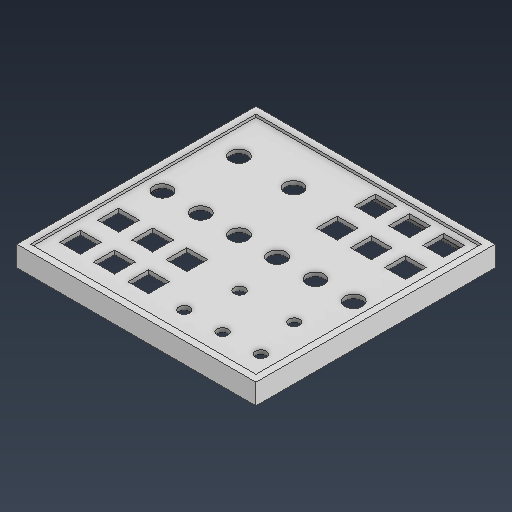
# Autodesk Inventor part: Faceplate
Saved by Autodesk Inventor 2025.3 (Build 293356000, 356)
## iProperties
Created: 2025-09-08
Part Number: Faceplate
Material: Generic
Document SubType Name: Modeling
Designer: tolga
Density: 1 g/cm^3
Appearance: Default
Author: tolga
Autodesk Inventor part; units mm, degrees
ref_plane "YZ Plane" through (0, 0, 0) normal (1, 0, 0) x (0, 1, 0)
ref_plane "XZ Plane" through (0, 0, 0) normal (0, 1, 0) x (-1, 0, 0)
ref_plane "XY Plane" through (0, 0, 0) normal (0, 0, 1) x (1, 0, 0)
sketch "Sketch1" plane through (0, 0, 0) normal (0, 1, 0) x (-1, 0, 0)
  line L0 (0, 0) -> (-175, 0)
  line L1 (-175, 0) -> (-175, -175)
  line L2 (-175, -175) -> (0, -175)
  line L3 (0, -175) -> (0, 0)
  dimension "d0" = 175
  dimension "d1" = 175
  constraints: 8 end point, 2 parallel, 1 horizontal, 1 perpendicular
  measures "d0" distance of L2.end L1.end
  measures "d1" distance of L1.end L0.end
extrude "Extrusion1" add sketch "Sketch1" along normal blind 3
sketch "Sketch2" plane through (0, 3, 0) normal (0, 1, 0) x (1, 0, 0)
  line L0 (175, 0) -> (175, 175) projected
  line L1 (175, 175) -> (0, 175) projected
  line L2 (0, 175) -> (0, 0) projected
  line L3 (0, 0) -> (175, 0) projected
  line L4 (5, 5) -> (5, 170)
  line L5 (5, 170) -> (170, 170)
  line L6 (170, 170) -> (170, 5)
  line L7 (170, 5) -> (5, 5)
  dimension "d4" = 5
  constraints: 8 end point, 3 other
  measures "d4" distance between parallel lines of L2 L4
extrude "Extrusion2" add sketch "Sketch2" along normal blind 2
sketch "Sketch3" plane through (0, 3, 0) normal (0, 1, 0) x (1, 0, 0)
  line L0 (5, 5) -> (170, 5) construction
  line L1 (170, 5) -> (170, 170) construction
  line L2 (170, 170) -> (5, 170) construction
  line L3 (5, 170) -> (5, 5) construction
  line L4 (6, 66) -> (84, 66) construction
  line L5 (84, 66) -> (84, 6) construction
  line L6 (84, 6) -> (6, 6) construction
  line L7 (6, 6) -> (6, 66) construction
  line L8 (91, 109) -> (169, 109) construction
  line L9 (169, 109) -> (169, 169) construction
  line L10 (169, 169) -> (91, 169) construction
  line L11 (91, 169) -> (91, 109) construction
  line L12 (6, 169) -> (81, 169) construction
  line L13 (81, 169) -> (81, 104) construction
  line L14 (6, 74) -> (6, 169) construction
  line L15 (6, 74) -> (169, 74) construction
  line L16 (169, 74) -> (169, 104) construction
  line L17 (169, 104) -> (81, 104) construction
  line L18 (89, 69) -> (169, 69) construction
  line L19 (169, 69) -> (169, 39) construction
  line L20 (169, 39) -> (89, 39) construction
  line L21 (89, 39) -> (89, 69) construction
  line L22 (89, 34) -> (169, 34) construction
  line L23 (169, 34) -> (169, 9) construction
  line L24 (169, 9) -> (89, 9) construction
  line L25 (89, 9) -> (89, 34) construction
  line L26 (12.4, 34) -> (27.6, 34)
  line L27 (27.6, 34) -> (27.6, 18.8)
  line L28 (27.6, 18.8) -> (12.4, 18.8)
  line L29 (12.4, 18.8) -> (12.4, 34)
  line L30 (12.4, 62) -> (27.6, 62)
  line L31 (12.4, 46.8) -> (12.4, 62)
  line L32 (27.6, 46.8) -> (12.4, 46.8)
  line L33 (27.6, 62) -> (27.6, 46.8)
  line L34 (37.4, 34) -> (52.6, 34)
  line L35 (37.4, 18.8) -> (37.4, 34)
  line L36 (52.6, 18.8) -> (37.4, 18.8)
  line L37 (52.6, 34) -> (52.6, 18.8)
  line L38 (37.4, 62) -> (52.6, 62)
  line L39 (37.4, 46.8) -> (37.4, 62)
  line L40 (52.6, 46.8) -> (37.4, 46.8)
  line L41 (52.6, 62) -> (52.6, 46.8)
  line L42 (62.4, 34) -> (77.6, 34)
  line L43 (62.4, 18.8) -> (62.4, 34)
  line L44 (77.6, 18.8) -> (62.4, 18.8)
  line L45 (77.6, 34) -> (77.6, 18.8)
  line L46 (62.4, 62) -> (77.6, 62)
  line L47 (62.4, 46.8) -> (62.4, 62)
  line L48 (77.6, 46.8) -> (62.4, 46.8)
  line L49 (77.6, 62) -> (77.6, 46.8)
  line L50 (12.4, 62) -> (12.4, 18.8) construction
  line L51 (12.4, 62) -> (77.6, 62) construction
  line L52 (97.4, 137) -> (112.6, 137)
  line L53 (112.6, 137) -> (112.6, 121.8)
  line L54 (112.6, 121.8) -> (97.4, 121.8)
  line L55 (97.4, 121.8) -> (97.4, 137)
  line L56 (97.4, 165) -> (112.6, 165)
  line L57 (97.4, 149.8) -> (97.4, 165)
  line L58 (112.6, 149.8) -> (97.4, 149.8)
  line L59 (112.6, 165) -> (112.6, 149.8)
  line L60 (122.4, 137) -> (137.6, 137)
  line L61 (122.4, 121.8) -> (122.4, 137)
  line L62 (137.6, 121.8) -> (122.4, 121.8)
  line L63 (137.6, 137) -> (137.6, 121.8)
  line L64 (122.4, 165) -> (137.6, 165)
  line L65 (122.4, 149.8) -> (122.4, 165)
  line L66 (137.6, 149.8) -> (122.4, 149.8)
  line L67 (137.6, 165) -> (137.6, 149.8)
  line L68 (147.4, 137) -> (162.6, 137)
  line L69 (147.4, 121.8) -> (147.4, 137)
  line L70 (162.6, 121.8) -> (147.4, 121.8)
  line L71 (162.6, 137) -> (162.6, 121.8)
  line L72 (147.4, 165) -> (162.6, 165)
  line L73 (147.4, 149.8) -> (147.4, 165)
  line L74 (162.6, 149.8) -> (147.4, 149.8)
  line L75 (162.6, 165) -> (162.6, 149.8)
  line L76 (97.4, 165) -> (97.4, 121.8) construction
  line L77 (97.4, 165) -> (162.6, 165) construction
  circle A0 centre (109, 54) radius 12.5 construction
  circle A1 centre (149, 54) radius 12.5 construction
  circle A2 centre (109, 54) radius 4
  circle A3 centre (149, 54) radius 4
  circle A4 centre (101, 21.5) radius 8.1 construction
  circle A5 centre (129, 21.5) radius 8.1 construction
  circle A6 centre (157, 21.5) radius 8.1 construction
  circle A7 centre (101, 21.5) radius 4
  circle A8 centre (129, 21.5) radius 4
  circle A9 centre (157, 21.5) radius 4
  circle A10 centre (157.5, 89) radius 6.5
  circle A11 centre (129.5, 89) radius 6.5
  circle A12 centre (101.5, 89) radius 6.5
  circle A13 centre (73.5, 89) radius 6.5
  circle A14 centre (45.5, 89) radius 6.5
  circle A15 centre (17.5, 89) radius 6.5
  circle A16 centre (63.5, 139) radius 6.5
  circle A17 centre (23.5, 139) radius 6.5
  point P0 (0, 0)
  point P1 (6, 36)
  point P2 (45, 62)
  point P3 (45, 66)
  point P4 (20, 46.8)
  point P5 (27.6, 54.4)
  point P6 (130, 165)
  point P7 (105, 149.8)
  point P8 (112.6, 157.4)
  point P9 (130, 165)
  point P10 (130, 109)
  point P11 (89, 54)
  point P12 (169, 21.5)
  point P13 (169, 89)
  point P14 (81, 136.5)
  dimension "d7" = 1
  dimension "d8" = 1
  dimension "d9" = 60
  dimension "d10" = 78
  dimension "d11" = 78
  dimension "d12" = 60
  dimension "d13" = 1
  dimension "d14" = 1
  dimension "d15" = 1
  dimension "d16" = 1
  dimension "d17" = 75
  dimension "d19" = 1
  dimension "d20" = 5
  dimension "d21" = 30
  dimension "d22" = 5
  dimension "d23" = 5
  dimension "d24" = 1
  dimension "d27" = 5
  dimension "d28" = 5
  dimension "d29" = 1
  dimension "d30" = 4
  dimension "d31" = 25
  dimension "d32" = 15.2
  dimension "d33" = 15.2
  dimension "d37" = 28
  dimension "d40" = 25
  dimension "d43" = 12.8
  dimension "d44" = 6.4
  dimension "d45" = 4
  dimension "d46" = 14
  dimension "d47" = 11.6
  dimension "d52" = 15.2
  dimension "d53" = 15.2
  dimension "d54" = 28
  dimension "d55" = 25
  dimension "d56" = 12.8
  dimension "d57" = 30
  dimension "d58" = 80
  dimension "d59" = 25
  dimension "d60" = 25
  dimension "d61" = 20
  dimension "d62" = 40
  dimension "d63" = 8
  dimension "d64" = 8
  dimension "d67" = 80
  dimension "d68" = 16.2
  dimension "d69" = 16.2
  dimension "d70" = 16.2
  dimension "d71" = 28
  dimension "d72" = 28
  dimension "d73" = 12
  dimension "d74" = 8
  dimension "d75" = 8
  dimension "d76" = 8
  dimension "d77" = 13
  dimension "d80" = 28
  dimension "d85" = 11.5
  dimension "d86" = 163
  dimension "d87" = 65
  dimension "d88" = 95
  dimension "d89" = 88
  dimension "d90" = 13
  dimension "d91" = 13
  dimension "d92" = 30
  constraints: 148 end point, 18 centre point, 14 midpoint, 13 parallel, 11 horizontal, 11 perpendicular, 7 horizontal alignment, 6 collinear, 5 coincident, 2 vertical, 2 vertical alignment, 86 other
  measures "d7" distance between parallel lines of L7 L3
  measures "d8" distance between parallel lines of L0 L6
  measures "d9" distance between parallel lines of L6 L4
  measures "d10" distance between parallel lines of L7 L5
  measures "d11" distance of L10.end L9.end
  measures "d12" distance of L9.end L8.end
  measures "d13" distance between parallel lines of L2 L10
  measures "d14" distance between parallel lines of L1 L9
  measures "d15" distance between parallel lines of L2 L12
  measures "d16" distance between parallel lines of L3 L14
  measures "d17" distance between parallel lines of L14 L13
  measures "d19" distance between parallel lines of L1 L16
  measures "d20" distance between parallel lines of L8 L17
  measures "d21" distance between parallel lines of L17 L15
  measures "d22" distance between parallel lines of L15 L18
  measures "d23" distance between parallel lines of L5 L21
  measures "d24" distance between parallel lines of L1 L19
  measures "d27" distance between parallel lines of L5 L25
  measures "d28" distance between parallel lines of L20 L22
  measures "d29" distance between parallel lines of L1 L23
  measures "d30" distance between parallel lines of L0 L24
  measures "d31" distance between parallel lines of L24 L22
  measures "d32" distance of L27.end L28.end
  measures "d33" distance of L26.end L27.end
  measures "d37" distance of L27.end L32.start
  measures "d40" distance of L27.end L36.start
  measures "d43" distance between parallel lines of L6 L28
  measures "d44" distance between parallel lines of L7 L31
  measures "d45" distance between parallel lines of L4 L51
  measures "d46" distance from line of L7 point (20, 46.8)
  measures "d47" distance from line of L4 point (27.6, 54.4)
  measures "d52" distance of L53.end L76.end
  measures "d53" distance of L53.start L53.end
  measures "d54" distance of L53.end L58.start
  measures "d55" distance of L53.end L62.start
  measures "d56" distance between parallel lines of L8 L54
  measures "d57" distance between parallel lines of L18 L20
  measures "d58" distance between parallel lines of L19 L21
  measures "d59" diameter of A0
  measures "d60" diameter of A1
  measures "d61" distance from line of L21 A0.centre
  measures "d62" distance of A0.centre A1.centre
  measures "d63" diameter of A2
  measures "d64" diameter of A3
  measures "d67" distance between parallel lines of L23 L25
  measures "d68" diameter of A4
  measures "d69" diameter of A5
  measures "d70" diameter of A6
  measures "d71" distance of A5.centre A4.centre
  measures "d72" distance of A6.centre A5.centre
  measures "d73" distance from line of L25 A4.centre
  measures "d74" diameter of A7
  measures "d75" diameter of A8
  measures "d76" diameter of A9
  measures "d77" diameter of A10
  measures "d80" distance of A10.centre A11.centre
  measures "d85" distance from line of L16 A10.centre
  measures "d86" distance of L14.start L15.end
  measures "d87" distance of L12.end L13.end
  measures "d88" distance of L14.start L12.start
  measures "d89" distance of L16.end L13.end
  measures "d90" diameter of A16
  measures "d91" diameter of A17
  measures "d92" distance from line of L12 A17.centre
extrude "Extrusion3" cut sketch "Sketch3" against normal up to surface (3 mm away)
sketch "Sketch4" plane through (0, 0, 0) normal (0, -1, 0) x (1, 0, 0)
  line L0 (175, 0) -> (175, -175) projected
  line L1 (0, 0) -> (175, 0) projected
  line L2 (175, -175) -> (0, -175) projected
  line L3 (0, -175) -> (0, 0) projected
  line L4 (172.6, -172.6) -> (172.6, -2.4)
  line L5 (172.6, -2.4) -> (2.4, -2.4)
  line L6 (2.4, -2.4) -> (2.4, -172.6)
  line L7 (2.4, -172.6) -> (172.6, -172.6)
  dimension "d95" = 2.4
  constraints: 8 end point, 3 other
  measures "d95" distance between parallel lines of L0 L4
extrude "Extrusion4" add sketch "Sketch4" along normal blind 10
equation "\"d8\" = d7"
equation "\"d11\" = d10"
equation "\"d12\" = d9"
equation "\"d13\" = d7"
equation "\"d14\" = d7"
equation "\"d15\" = d7"
equation "\"d16\" = d7"
equation "\"d19\" = d7"
equation "\"d24\" = d7"
equation "\"d29\" = d7"
equation "\"d43\" = d37 - d33"
equation "\"d56\" = d43"
equation "\"d60\" = d59"
equation "\"d61\" = -0.5 * d62 + 0.5 * d58"
equation "\"d64\" = d63"
equation "\"d69\" = d68"
equation "\"d70\" = d68"
equation "\"d72\" = d71"
equation "\"d73\" = -d71 + 0.5 * d67"
equation "\"d75\" = d74"
equation "\"d76\" = d74"
body "Solid1"
